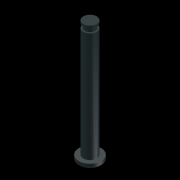
# Autodesk Inventor part: shaft6-47.8
Saved by Autodesk Inventor 2011 (Build 150239000, 239)
## iProperties
Created: 2013-02-08
Part Number: shaft6-47.8
Document SubType Name: Modeling
Designer: JohnHenry
Density: 1 g/cm^3
Author: JohnHenry
Autodesk Inventor part; units mm, degrees
ref_plane "YZ Plane" through (0, 0, 0) normal (1, 0, 0) x (0, 1, 0)
ref_plane "XZ Plane" through (0, 0, 0) normal (0, 1, 0) x (-1, 0, 0)
ref_plane "XY Plane" through (0, 0, 0) normal (0, 0, 1) x (1, 0, 0)
sketch "スケッチ1" plane through (0, 0, 0) normal (0, 0, 1) x (1, 0, 0)
  circle A0 centre (0, 0) radius 3
  dimension "d0" = 6
  constraints: 1 centre point, 1 coincident
  measures "d0" diameter of A0
extrude "押し出し1" add sketch "スケッチ1" along normal blind 47.8
sketch "スケッチ2" plane through (0, 0, 0) normal (0, 0, -1) x (-1, 0, 0)
  circle A0 centre (0, 0) radius 3 projected
  circle A1 centre (0, 0) radius 5
  dimension "d3" = 10
  constraints: 1 centre point, 1 coincident
  measures "d3" diameter of A1
extrude "押し出し2" add sketch "スケッチ2" along normal blind 2 contours A0 | A1
sketch "スケッチ3" plane through (0, 0, 47.8) normal (0, 0, 1) x (1, 0, 0)
  circle A0 centre (0, 0) radius 3 projected
extrude "押し出し3" add sketch "スケッチ3" along normal blind 1
sketch "スケッチ4" plane through (0, 0, 48.8) normal (0, 0, 1) x (1, 0, 0)
  circle A0 centre (0, 0) radius 3 projected
  circle A1 centre (0, 0) radius 2.25
  dimension "d8" = 4.5
  constraints: 1 centre point, 1 coincident
  measures "d8" diameter of A1
extrude "押し出し4" add sketch "スケッチ4" along normal blind 2 contours A1
sketch "スケッチ5" plane through (0, 0, 50.8) normal (0, 0, 1) x (1, 0, 0)
  circle A0 centre (0, 0) radius 2.25 projected
  circle A1 centre (0, 0) radius 3
  dimension "d11" = 6
  constraints: 1 centre point, 1 coincident
  measures "d11" diameter of A1
extrude "押し出し5" add sketch "スケッチ5" along normal blind 1 contours A0 | A1
chamfer "面取り1" distance 0.5 angle 45 1 edges at (5, 0, -2)
